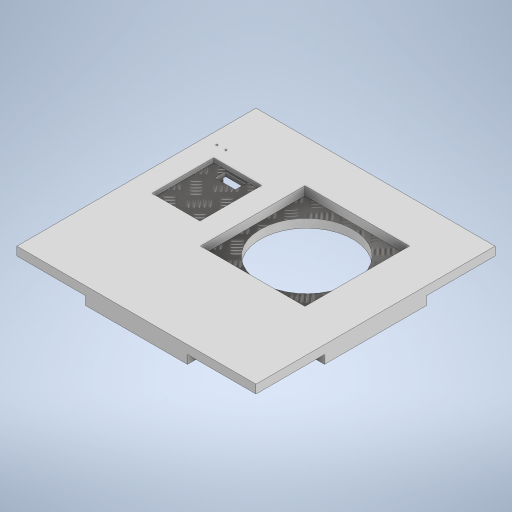
# Autodesk Inventor part: FinalBoxTop
Saved by Autodesk Inventor 2023 (Build 270158000, 158)
## iProperties
Created: 2023-09-21
Part Number: FinalBoxTop
Material: Generic
Document SubType Name: Modeling
Designer: Gage
Density: 1 g/cm^3
Appearance: Default
Author: Gage
## iProperties of the stored document FinalBoxTop_3DPrint.ipt
Created: 2023-09-28
Part Number: FinalBoxTop_3DPrint
Material: Generic
Document SubType Name: Modeling
Designer: Gage
Density: 1 g/cm^3
Appearance: Default
Author: Gage
Autodesk Inventor part; units mm, degrees
ref_plane "YZ Plane" through (0, 0, 0) normal (1, 0, 0) x (0, 1, 0)
ref_plane "XZ Plane" through (0, 0, 0) normal (0, 1, 0) x (-1, 0, 0)
ref_plane "XY Plane" through (0, 0, 0) normal (0, 0, 1) x (1, 0, 0)
sketch "Sketch1" plane through (0, 0, 0) normal (0, 1, 0) x (-1, 0, 0)
  line L0 (44.323, -44.323) -> (-44.323, -44.323)
  line L1 (-44.323, -44.323) -> (-44.323, 44.323)
  line L2 (-44.323, 44.323) -> (44.323, 44.323)
  line L3 (44.323, 44.323) -> (44.323, -44.323)
  point P0 (0, 0)
  point P1 (0, 44.323)
  point P2 (-44.323, 0)
  dimension "d0" = 88.646
  dimension "d1" = 88.646
  constraints: 8 end point, 2 midpoint, 2 parallel, 1 horizontal, 1 horizontal alignment, 1 perpendicular, 1 vertical alignment
  measures "d0" distance of L1.end L2.end
  measures "d1" distance of L0.end L1.end
extrude "Extrusion1" add sketch "Sketch1" along normal blind 6.35
sketch "Sketch2" plane through (0, 0, 0) normal (0, -1, 0) x (1, 0, 0)
  line L0 (-44.323, 44.323) -> (44.323, 44.323) projected
  line L1 (-44.323, 44.323) -> (-18.923, 44.323)
  line L2 (-18.923, 44.323) -> (-18.923, 18.923)
  line L3 (-18.923, 18.923) -> (-44.323, 18.923)
  line L4 (-44.323, 18.923) -> (-44.323, 44.323)
  line L5 (44.323, 44.323) -> (18.923, 44.323)
  line L6 (18.923, 44.323) -> (18.923, 18.923)
  line L7 (18.923, 18.923) -> (44.323, 18.923)
  line L8 (44.323, 18.923) -> (44.323, 44.323)
  line L9 (44.323, 44.323) -> (44.323, -44.323) projected
  line L10 (44.323, -44.323) -> (18.923, -44.323)
  line L11 (18.923, -44.323) -> (18.923, -18.923)
  line L12 (18.923, -18.923) -> (44.323, -18.923)
  line L13 (44.323, -18.923) -> (44.323, -44.323)
  line L14 (44.323, -44.323) -> (-44.323, -44.323) projected
  line L15 (-44.323, -44.323) -> (-18.923, -44.323)
  line L16 (-18.923, -44.323) -> (-18.923, -18.923)
  line L17 (-18.923, -18.923) -> (-44.323, -18.923)
  line L18 (-44.323, -18.923) -> (-44.323, -44.323)
  line L19 (44.323, -44.323) -> (28.448, -44.323)
  line L20 (28.448, -44.323) -> (28.448, -28.448)
  line L21 (28.448, -28.448) -> (44.323, -28.448)
  line L22 (44.323, -28.448) -> (44.323, -44.323)
  line L23 (28.448, -28.448) -> (28.448, -18.923)
  line L24 (28.448, -28.448) -> (18.923, -28.575)
  point P0 (0, 0)
  point P1 (44.323, -18.923)
  dimension "d4" = 25.4
  dimension "d5" = 25.4
  dimension "d6" = 25.4
  dimension "d7" = 25.4
  dimension "d8" = 25.4
  dimension "d9" = 25.4
  dimension "d10" = 25.4
  dimension "d11" = 25.4
  dimension "d147" = 15.875
  dimension "d148" = 15.875
  constraints: 44 end point, 10 parallel, 6 perpendicular, 5 horizontal, 2 point on line
  measures "d4" distance of L2.end L3.end
  measures "d5" distance of L1.end L2.end
  measures "d6" distance of L7.end L6.end
  measures "d7" distance of L6.end L5.end
  measures "d8" distance of L11.end L12.end
  measures "d9" distance of L10.end L11.end
  measures "d10" distance of L17.end L16.end
  measures "d11" distance of L16.end L15.end
  measures "d147" distance of L20.end L21.end
  measures "d148" distance of L19.end L20.end
extrude "Extrusion2" cut sketch "Sketch2" against normal blind 3.175 contours L0 L2 L3 L4 | L0 L8 L7 L6 | L9 L21 L23 L12 | L9 L10 L20 L21 | L20 L10 L11 L24 | L14 L18 L17 L16
sketch "Sketch3" plane through (0, 6.35, 0) normal (0, 1, 0) x (1, 0, 0)
  line L0 (-45.72, 45.72) -> (45.72, 45.72)
  line L1 (45.72, 45.72) -> (45.72, -45.72)
  line L2 (45.72, -45.72) -> (-45.72, -45.72)
  line L3 (-45.72, -45.72) -> (-45.72, 45.72)
  point P0 (0, 0)
  point P1 (45.72, 0)
  point P2 (0, 45.72)
  dimension "d14" = 91.44
  dimension "d15" = 91.44
  constraints: 8 end point, 2 midpoint, 2 parallel, 1 horizontal, 1 horizontal alignment, 1 perpendicular, 1 vertical alignment
  measures "d14" distance of L1.end L2.end
  measures "d15" distance of L0.end L1.end
extrude "Extrusion3" [suppressed]
sketch "Sketch4" plane through (0, 3.175, 0) normal (0, -1, 0) x (1, 0, 0)
  circle A0 centre (-38.1, 38.1) radius 3.175
  circle A1 centre (38.1, 38.1) radius 3.175
  circle A2 centre (38.1, -38.1) radius 3.175
  circle A3 centre (-38.1, -38.1) radius 3.175
  line L0 (44.323, 44.323) -> (44.323, 18.923) projected
  line L1 (18.923, 44.323) -> (44.323, 44.323) projected
  line L2 (-44.323, 44.323) -> (-18.923, 44.323) projected
  line L3 (-44.323, 18.923) -> (-44.323, 44.323) projected
  line L4 (-44.323, -44.323) -> (-44.323, -18.923) projected
  line L5 (-18.923, -44.323) -> (-44.323, -44.323) projected
  line L6 (44.323, -18.923) -> (44.323, -44.323) projected
  line L7 (44.323, -44.323) -> (18.923, -44.323) projected
  point P0 (0, 0)
  point P1 (44.323, 31.623)
  point P2 (-31.623, 44.323)
  point P3 (-44.323, -31.623)
  point P4 (44.323, -31.623)
  point P5 (31.623, -44.323)
  dimension "d19" = 6.35
  dimension "d20" = 6.35
  dimension "d21" = 6.35
  dimension "d22" = 6.35
  dimension "d23" = 6.223
  dimension "d24" = 6.223
  dimension "d25" = 6.223
  dimension "d26" = 6.223
  dimension "d27" = 6.223
  dimension "d28" = 6.223
  dimension "d29" = 6.223
  dimension "d30" = 6.223
  constraints: 5 midpoint, 4 centre point
  measures "d19" diameter of A0
  measures "d20" diameter of A1
  measures "d21" diameter of A2
  measures "d22" diameter of A3
  measures "d23" horizontal distance of point (44.323, 31.623) A1.centre
  measures "d24" distance from line of L1 A1.centre
  measures "d25" vertical distance of point (-31.623, 44.323) A0.centre
  measures "d26" distance from line of L3 A0.centre
  measures "d27" horizontal distance of point (-44.323, -31.623) A3.centre
  measures "d28" distance from line of L5 A3.centre
  measures "d29" horizontal distance of point (44.323, -31.623) A2.centre
  measures "d30" vertical distance of point (31.623, -44.323) A2.centre
extrude "Extrusion4" [suppressed]
sketch "Sketch5" plane through (0, 9.525, 0) normal (0, 1, 0) x (1, 0, 0)
  line L0 (44.323, 44.323) -> (-44.323, 44.323) projected
  line L1 (44.323, 44.323) -> (28.448, 44.323)
  line L2 (28.448, 44.323) -> (28.448, 28.448)
  line L3 (28.448, 28.448) -> (44.323, 28.448)
  line L4 (44.323, 28.448) -> (44.323, 44.323)
  line L5 (28.448, 28.448) -> (-10.287, 28.448)
  line L6 (-10.287, 28.448) -> (-10.287, -10.287)
  line L7 (-10.287, -10.287) -> (28.448, -10.287)
  line L8 (28.448, -10.287) -> (28.448, 28.448)
  line L9 (-10.287, 28.448) -> (-1.397, 28.448)
  line L10 (-1.397, 28.448) -> (-1.397, 22.6515)
  line L11 (-4.4905, 19.558) -> (-10.287, 19.558)
  line L12 (-10.287, 19.558) -> (-10.287, 28.448)
  line L13 (28.448, 28.448) -> (19.558, 28.448)
  line L14 (19.558, 28.448) -> (19.558, 22.6515)
  line L15 (22.6515, 19.558) -> (28.448, 19.558)
  line L16 (28.448, 19.558) -> (28.448, 28.448)
  line L17 (28.448, -10.287) -> (19.558, -10.287)
  line L18 (19.558, -10.287) -> (19.558, -4.4905)
  line L19 (22.6515, -1.397) -> (28.448, -1.397)
  line L20 (28.448, -1.397) -> (28.448, -10.287)
  line L21 (-10.287, -10.287) -> (-1.397, -10.287)
  line L22 (-1.397, -10.287) -> (-1.397, -4.4905)
  line L23 (-4.4905, -1.397) -> (-10.287, -1.397)
  line L24 (-10.287, -1.397) -> (-10.287, -10.287)
  circle A0 centre (9.0805, 9.0805) radius 17.145
  point P0 (0, 0)
  point P1 (19.558, -10.287)
  point P2 (28.448, -1.397)
  point P3 (-1.397, 28.448)
  point P4 (-10.287, 19.558)
  point P5 (-1.397, -4.4905)
  point P6 (19.558, -4.4905)
  point P7 (22.6515, -1.397)
  point P8 (-1.397, 22.6515)
  point P9 (-4.4905, 19.558)
  point P10 (-4.4905, -1.397)
  point P11 (28.448, 9.0805)
  point P12 (9.0805, 28.448)
  point P13 (-10.287, 24.003)
  point P14 (-5.842, -10.287)
  point P15 (-7.3888, -1.397)
  point P16 (28.448, 24.003)
  point P17 (19.558, 24.003)
  dimension "d125" = 34.29
  dimension "d33" = 15.875
  dimension "d34" = 15.875
  dimension "d35" = 38.735
  dimension "d36" = 38.735
  dimension "d126" = 8.89
  dimension "d127" = 8.89
  dimension "d128" = 8.89
  dimension "d129" = 8.89
  dimension "d130" = 8.89
  dimension "d131" = 8.89
  dimension "d132" = 8.89
  dimension "d133" = 8.89
  constraints: 48 end point, 12 parallel, 6 horizontal, 6 midpoint, 6 perpendicular, 1 horizontal alignment, 1 point on line, 1 vertical alignment, 10 other
  measures "d33" distance of L3.end L2.end
  measures "d34" distance of L2.end L1.end
  measures "d35" distance of L7.end L6.end
  measures "d36" distance of L6.end L5.end
  measures "d126" distance between parallel lines of L5 L11
  measures "d127" distance from line of L10 point (-10.287, 24.003)
  measures "d128" vertical distance of point (-5.842, -10.287) point (-7.389, -1.397)
  measures "d129" distance between parallel lines of L6 L22
  measures "d130" distance between parallel lines of L17 L19
  measures "d131" distance between parallel lines of L18 L8
  measures "d132" distance of point (28.448, 24.003) point (19.558, 24.003)
  measures "d133" distance between parallel lines of L5 L15
extrude "Extrusion5" [suppressed]
sketch "Sketch7" plane through (0, 9.525, 0) normal (0, 1, 0) x (1, 0, 0)
  line L0 (44.323, -44.323) -> (44.323, 44.323) projected
  line L1 (44.323, 44.323) -> (28.448, 44.323)
  line L2 (28.448, 44.323) -> (28.448, 28.448)
  line L3 (28.448, 28.448) -> (44.323, 28.448)
  line L4 (44.323, 28.448) -> (44.323, 44.323)
  line L5 (28.448, 28.448) -> (-10.287, 28.448)
  line L6 (-10.287, 28.448) -> (-10.287, -10.287)
  line L7 (-10.287, -10.287) -> (28.448, -10.287)
  line L8 (28.448, -10.287) -> (28.448, 28.448)
  line L9 (-10.287, 28.448) -> (-1.397, 28.448)
  line L10 (-10.287, 19.558) -> (-10.287, 28.448)
  line L11 (28.448, 28.448) -> (19.558, 28.448)
  line L12 (28.448, 19.558) -> (28.448, 28.448)
  line L13 (28.448, -10.287) -> (19.558, -10.287)
  line L14 (28.448, -1.397) -> (28.448, -10.287)
  line L15 (-10.287, -10.287) -> (-1.397, -10.287)
  line L16 (-10.287, -1.397) -> (-10.287, -10.287)
  point P0 (0, 0)
  point P1 (-1.397, 28.448)
  dimension "d62" = 15.875
  dimension "d63" = 15.875
  dimension "d64" = 38.735
  dimension "d65" = 38.735
  constraints: 32 end point, 6 horizontal, 4 parallel, 2 perpendicular
  measures "d62" distance of L3.end L2.end
  measures "d63" distance of L1.end L2.end
  measures "d64" distance of L7.end L6.end
  measures "d65" distance of L6.end L5.end
extrude "Extrusion7" [suppressed]
sketch "Sketch9" plane through (0, 9.525, 0) normal (0, 1, 0) x (1, 0, 0)
  point P0 (0, 0)
sketch "Sketch11" plane through (0, 9.525, 0) normal (0, 1, 0) x (1, 0, 0)
  point P0 (0, 0)
sketch "Sketch12" plane through (0, 0, 0) normal (0, -1, 0) x (1, 0, 0)
  line L0 (18.923, -44.323) -> (-31.75, -44.323)
  line L1 (-31.75, -44.323) -> (-31.75, -42.545)
  line L2 (18.923, -55.245) -> (18.923, -44.323)
  line L3 (-31.75, -42.545) -> (16263.8032, -42.545)
  line L4 (16263.8032, -42.545) -> (16263.8032, -31.623)
  line L5 (16263.8032, -31.623) -> (-31.75, -31.623)
  line L6 (-31.75, -31.623) -> (-31.75, -42.545)
  line L7 (-44.323, -18.923) -> (-44.323, 18.923) projected
  line L8 (16263.8032, -31.623) -> (-44.323, -31.623)
  line L9 (-44.323, -31.623) -> (-44.323, -30.0228)
  line L10 (-44.323, -30.0228) -> (16263.8032, -30.0228)
  line L11 (16263.8032, -30.0228) -> (16263.8032, -31.623)
  line L12 (-18.923, 18.923) -> (-44.323, 18.923) projected
  line L13 (-44.323, -30.0228) -> (-42.7228, -30.0228)
  line L14 (-42.7228, -30.0228) -> (-42.7228, 18.923)
  line L15 (-42.7228, 18.923) -> (-44.323, 18.923)
  line L16 (-44.323, 18.923) -> (-44.323, -30.0228)
  line L17 (-42.7228, 18.923) -> (-31.7277, 18.923)
  line L18 (-31.7277, 18.923) -> (-31.7277, 180.443)
  line L19 (-31.7277, 180.443) -> (-42.7228, 180.443)
  line L20 (-42.7228, 180.443) -> (-42.7228, 18.923)
  line L21 (-18.923, 44.323) -> (18.923, 44.323) projected
  line L22 (-31.7277, 180.443) -> (-30.1275, 180.443)
  line L23 (-30.1275, 180.443) -> (-30.1275, 44.323)
  line L24 (-30.1275, 44.323) -> (-31.7277, 44.323)
  line L25 (-31.7277, 44.323) -> (-31.7277, 180.443)
  line L26 (18.923, 18.923) -> (18.923, 44.323) projected
  line L27 (-30.1275, 44.323) -> (18.923, 44.323)
  line L28 (18.923, 44.323) -> (18.923, 42.7228)
  line L29 (18.923, 42.7228) -> (-30.1275, 42.7228)
  line L30 (-30.1275, 42.7228) -> (-30.1275, 44.323)
  line L31 (18.923, 42.7228) -> (17.3228, 42.7228)
  line L32 (17.3228, 42.7228) -> (17.3228, 18.923)
  line L33 (17.3228, 18.923) -> (18.923, 18.923)
  line L34 (18.923, 18.923) -> (18.923, 42.7228)
  line L35 (44.323, 44.323) -> (44.323, -44.323) projected
  line L36 (17.3228, 18.923) -> (44.323, 18.923)
  line L37 (44.323, 18.923) -> (44.323, 180.443)
  line L38 (44.323, 180.443) -> (17.3228, 180.443)
  line L39 (17.3228, 180.443) -> (17.3228, 18.923)
  line L40 (28.448, -18.923) -> (44.323, -18.923) projected
  line L41 (44.323, 180.443) -> (42.7228, 180.443)
  line L42 (42.7228, 180.443) -> (42.7228, -18.923)
  line L43 (42.7228, -18.923) -> (44.323, -18.923)
  line L44 (44.323, -18.923) -> (44.323, 180.443)
  line L45 (42.7228, -18.923) -> (18.923, -18.923)
  line L46 (18.923, -18.923) -> (18.923, -24.2084)
  line L47 (18.923, -24.2084) -> (42.7228, -24.2084)
  line L48 (42.7228, -24.2084) -> (42.7228, -18.923)
  line L49 (18.923, -24.2084) -> (17.3228, -24.2084)
  line L50 (17.3228, -24.2084) -> (17.3228, -42.545)
  line L51 (17.3228, -42.545) -> (18.923, -42.545)
  line L52 (18.923, -42.545) -> (18.923, -24.2084)
  line L53 (18.923, -44.323) -> (18.923, -28.575) projected
  line L54 (-18.923, -18.923) -> (-18.923, -44.323) projected
  line L55 (18.923, -44.323) -> (-18.923, -44.323)
  line L56 (-18.923, -44.323) -> (-18.923, -42.7228)
  line L57 (-18.923, -42.7228) -> (18.923, -42.7228)
  line L58 (18.923, -42.7228) -> (18.923, -44.323)
  line L59 (17.3228, -42.545) -> (18.923, -42.545)
  line L60 (18.923, -42.545) -> (18.923, -42.7228)
  line L61 (18.923, -42.7228) -> (17.3228, -42.7228)
  line L62 (17.3228, -42.7228) -> (17.3228, -42.545)
  line L63 (16263.8032, -42.545) -> (-18.923, -42.545)
  line L64 (-18.923, -42.545) -> (-18.923, -42.7228)
  line L65 (-18.923, -42.7228) -> (16263.8032, -42.7228)
  line L66 (16263.8032, -42.7228) -> (16263.8032, -42.545)
  line L67 (-10.287, -28.448) -> (28.448, -28.448) projected
  line L68 (-9.525, 9.525) -> (28.448, 9.525)
  line L69 (28.448, 9.525) -> (28.448, -28.448)
  line L70 (28.448, -28.448) -> (-9.525, -28.448)
  line L71 (-9.525, -28.448) -> (-9.525, 9.525)
  line L72 (17.3228, -24.2084) -> (-5.867, -24.2084)
  line L73 (-5.867, -24.2084) -> (-5.867, 154.3887)
  line L74 (-5.867, 154.3887) -> (17.3228, 154.3887)
  line L75 (17.3228, 154.3887) -> (17.3228, -24.2084)
  line L76 (17.3228, -24.2084) -> (-1.1916, -42.7228)
  line L77 (17.3228, -24.2084) -> (49.6283, -24.2084) construction
  line L78 (-1.1916, -42.7228) -> (-19.7059, -24.2084)
  line L79 (-1.1916, -42.7228) -> (35.5335, -42.7228) construction
  line L80 (-19.7059, -24.2084) -> (-32.8283, -42.7228)
  line L81 (-32.8283, -42.7228) -> (-42.7228, -35.7099)
  line L82 (-42.7228, -35.7099) -> (12.8674, 42.7228)
  line L83 (12.8674, 42.7228) -> (42.7228, 63.8728)
  line L84 (42.7228, 63.8728) -> (17.3228, 28.0357)
  line L85 (17.3228, 28.0357) -> (42.7228, 10.0331)
  line L86 (42.7228, 10.0331) -> (17.3228, -25.8039)
  line L87 (17.4453, -24.2084) -> (-2.7918, -42.7228)
  line L88 (-2.7918, -42.7228) -> (-19.7301, -24.2084)
  line L89 (-19.7301, -24.2084) -> (-39.9672, -42.7228)
  line L90 (-39.9672, -42.7228) -> (-42.7228, -39.7108)
  line L91 (-42.7228, -39.7108) -> (39.9672, 35.94)
  line L92 (39.9672, 35.94) -> (42.7228, 32.928)
  line L93 (42.7228, 32.928) -> (17.3228, 9.6902)
  line L94 (17.3228, 9.6902) -> (42.7228, -1.0828)
  line L95 (42.7228, -1.0828) -> (17.3228, -24.3205)
  line L96 (17.3228, -42.7228) -> (17.1896, -24.2084)
  line L97 (17.1896, -24.2084) -> (4.3578, -42.7228)
  line L98 (4.3578, -42.7228) -> (-22.3557, -24.2084)
  line L99 (-22.3557, -24.2084) -> (-35.0642, -42.545)
  line L100 (-42.545, -42.545) -> (42.545, -42.545) projected
  line L101 (-35.0642, -42.545) -> (16263.8032, -11338.832)
  line L102 (16263.8032, -11338.832) -> (-5.867, -34813.5541)
  line L103 (-5.867, -34813.5541) -> (-42.7228, -34788.0104)
  line L104 (-42.7228, -34788.0104) -> (24192.9295, 180.443)
  line L105 (42.7228, -24.2084) -> (17.3228, -17.3228)
  line L106 (17.3228, -17.3228) -> (42.7228, 76.3738)
  line L107 (42.7228, 76.3738) -> (17.3228, 83.2595)
  line L108 (17.3228, 83.2595) -> (42.7228, 176.9561)
  line L109 (42.7228, 176.9561) -> (29.8603, 180.443)
  line L110 (29.8603, 180.443) -> (22.7974, 154.3887)
  line L111 (42.7228, -22.6082) -> (17.3228, -15.7226)
  line L112 (17.3228, -15.7226) -> (42.7228, 77.974)
  line L113 (42.7228, 77.974) -> (17.3228, 84.8597)
  line L114 (17.3228, 84.8597) -> (42.7228, 22.3774)
  line L115 (42.7228, 22.3774) -> (431.5533, 180.443)
  line L116 (431.5533, 180.443) -> (442.1447, 154.3887)
  line L117 (15.7226, -42.7228) -> (15.5894, -24.2084)
  line L118 (15.5894, -24.2084) -> (-2558.3431, -42.7228)
  line L119 (-2558.3431, -42.7228) -> (-2558.4763, -24.2084)
  line L120 (-2558.4763, -24.2084) -> (-5132.4088, -42.7228)
  line L121 (-5132.4088, -42.7228) -> (-5095.6192, -5157.3332)
  line L122 (-5095.6192, -5157.3332) -> (-5.867, -5120.7225)
  line L123 (-5.867, -5120.7225) -> (-42.7228, 3.0988)
  line L124 (-42.7228, 3.0988) -> (5465.9431, 42.7228)
  line L125 (24192.9295, 180.443) -> (5046.5957, 42.7228)
  line L126 (5046.5957, 42.7228) -> (22.7974, 154.3887)
  line L127 (442.1447, 154.3887) -> (5465.9431, 42.7228)
  line L128 (-5.867, 154.3887) -> (-42.545, -32.2271)
  line L129 (-42.545, 42.545) -> (-42.545, -42.545) projected
  line L130 (-42.545, -32.2271) -> (-42.7228, -33.1317)
  line L131 (-42.7228, -33.1317) -> (-42.7228, -31.5315)
  line L132 (-42.7228, -31.5315) -> (6.1315, 42.7228)
  line L133 (-5.867, 154.3887) -> (-79.3356, 42.7228)
  line L134 (17.3228, -42.545) -> (16263.8032, -42.545)
  line L135 (-42.545, -30.0228) -> (-42.545, 180.443)
  point P0 (0, 0)
  point P1 (18.923, -18.923)
  point P2 (19.558, -28.448)
  point P3 (17.3228, -15.7226)
  point P4 (17.7269, -15.8321)
  point P5 (24.5726, -17.6879)
  point P6 (41.9227, -16.5227)
  point P7 (27.6372, 20.7253)
  point P8 (23.8906, 6.9046)
  point P9 (23.3165, -17.3474)
  point P10 (23.2233, -18.9223)
  point P11 (27.2733, 20.9832)
  point P12 (35.5727, 2.5273)
  point P13 (17.7269, 84.7501)
  point P14 (36.3728, 3.3274)
  point P15 (41.9227, 8.8773)
  point P16 (36.3728, 14.4272)
  point P17 (23.5015, 7.0696)
  point P18 (42.3187, 76.4834)
  point P19 (36.3728, 1.7272)
  point P20 (30.8229, -3.8227)
  point P21 (37.1729, 2.5273)
  point P22 (37.1729, 15.2273)
  point P23 (34.0995, 29.4005)
  point P24 (28.5496, 23.8506)
  point P25 (36.3728, 16.0274)
  point P26 (41.9227, 21.5773)
  point P27 (27.7495, 23.0505)
  point P28 (29.6259, 54.5948)
  point P29 (14.2544, 38.1458)
  point P30 (9.6774, 42.7228)
  point P31 (15.0545, 37.3457)
  point P32 (27.7495, 24.6507)
  point P33 (14.2544, 36.5456)
  point P34 (2.2571, 24.5482)
  point P35 (15.0079, 11.9091)
  point P36 (26.9494, 23.8506)
  point P37 (1.4535, 25.3448)
  point P38 (13.4543, 37.3457)
  point P39 (8.8773, 41.9227)
  point P40 (-3.1437, 29.9017)
  point P41 (-3.9474, 30.6982)
  point P42 (-42.545, 30.2006)
  point P43 (-42.545, 17.8544)
  point P44 (-4.7439, 29.9017)
  point P45 (-16.8706, 41.9221)
  point P46 (-41.7927, 16.7387)
  point P47 (-29.9115, 4.7341)
  point P48 (-24.5621, -0.6708)
  point P49 (0.6569, 24.5482)
  point P50 (-3.9403, 29.1051)
  point P51 (-29.1155, 3.9299)
  point P52 (-42.545, -21.6196)
  point P53 (-42.545, -35.4591)
  point P54 (-42.4465, -35.32)
  point P55 (1.4605, 23.7516)
  point P56 (-23.7661, -1.475)
  point P57 (-42.545, -31.2613)
  point P58 (-38.1458, -14.2544)
  point P59 (-42.545, -39.9051)
  point P60 (-37.3457, -13.4543)
  point P61 (-42.4764, -31.157)
  point P62 (-42.4169, -39.4309)
  point P63 (-40.2587, -37.4564)
  point P64 (-24.7626, -27.6376)
  point P65 (-37.3457, -15.0545)
  point P66 (-42.4714, -31.8526)
  point P67 (-36.5456, -14.2544)
  point P68 (-23.9584, -26.8416)
  point P69 (-11.7974, -14.8056)
  point P70 (17.1913, -24.4408)
  point P71 (30.0228, -30.0228)
  point P72 (18.4536, -24.2084)
  point P73 (17.3228, -25.8039)
  point P74 (22.3651, -18.6897)
  point P75 (17.3215, -42.545)
  point P76 (17.1906, -24.3406)
  point P77 (15.7213, -42.545)
  point P78 (15.6018, -25.9294)
  point P79 (-1.0138, -42.545)
  point P80 (15.6016, -25.8952)
  point P81 (15.6059, -26.4936)
  point P82 (10.8738, -36.2738)
  point P83 (-1.9561, -41.9583)
  point P84 (4.4811, -42.545)
  point P85 (-2.9544, -42.545)
  point P86 (10.0695, -37.0697)
  point P87 (-19.4539, -24.4605)
  point P88 (-20.8618, -25.2438)
  point P89 (-21.9659, -24.4786)
  point P90 (-19.4992, -24.4608)
  point P91 (-19.7165, -24.2233)
  point P92 (-20.5788, -25.4399)
  point P93 (2.8416, -42.545)
  point P94 (-2.5569, -37.2025)
  point P95 (-32.7022, -42.545)
  point P96 (-40.1298, -42.545)
  point P97 (-15.3311, -37.0691)
  point P98 (-22.5598, -42.545)
  point P99 (-30.2464, -34.9382)
  point P100 (-24.0131, -28.3871)
  point P101 (-29.4444, -33.8754)
  point P102 (-21.5341, -41.8678)
  point P103 (-16.0619, -36.3383)
  point P104 (-23.2172, -27.5828)
  point P105 (-15.266, -35.534)
  point P106 (-3.3612, -36.4066)
  point P107 (-9.0118, -30.8147)
  point P108 (-34.4103, -41.6015)
  point P109 (-36.8508, -39.8717)
  dimension "d94" = 1.6002
  dimension "d95" = 1.6002
  dimension "d96" = 1.6002
  dimension "d97" = 1.6002
  dimension "d98" = 1.6002
  dimension "d99" = 1.6002
  dimension "d100" = 1.6002
  dimension "d101" = 1.6002
  dimension "d102" = 135
  dimension "d103" = 135
  dimension "d104" = 1.6002
  dimension "d105" = 1.6002
  dimension "d106" = 1.6002
  dimension "d107" = 1.6002
  dimension "d108" = 1.6002
  dimension "d109" = 1.6002
  dimension "d110" = 1.6002
  constraints: 240 end point, 46 perpendicular, 42 point on line, 31 parallel, 22 horizontal, 3 vertical, 49 other
  measures "d94" distance of L8.end L9.end
  measures "d95" distance of L15.end L14.end
  measures "d96" distance of L24.end L23.end
  measures "d97" distance of L27.end L28.end
  measures "d98" distance of L33.end L32.end
  measures "d99" distance of L43.end L43.start
  measures "d100" distance of L51.end L50.end
  measures "d101" distance of L55.end L56.end
  measures "d102" angle of L76 L77
  measures "d103" angle of L79 L78
  measures "d104" distance of L87.start L86.end
  measures "d105" distance of L87.end L76.end
  measures "d106" distance of point (17.323, -15.723) L105.end
  measures "d107" distance of L111.start L47.end
  measures "d108" distance of L117.end L96.end
  measures "d109" distance of L117.start L61.end
  measures "d110" distance of L130.end L131.end
extrude "Extrusion10" [suppressed]
sketch "Sketch13" plane through (0, 9.525, 0) normal (0, 1, 0) x (1, 0, 0)
  circle A0 centre (-39.6875, -28.575) radius 0.3175
  circle A1 centre (-36.3855, -28.575) radius 0.3175
  line L0 (-45.72, 45.72) -> (-45.72, -45.72) projected
  line L1 (-45.72, -45.72) -> (45.72, -45.72) projected
  point P0 (0, 0)
  dimension "d113" = 0.635
  dimension "d114" = 0.635
  dimension "d115" = 3.302
  dimension "d149" = 6.0325
  dimension "d150" = 17.145
  constraints: 2 centre point
  measures "d113" diameter of A0
  measures "d114" diameter of A1
  measures "d115" distance of A1.centre A0.centre
  measures "d149" distance from line of L0 A0.centre
  measures "d150" distance from line of L1 A0.centre
extrude "Extrusion11" [suppressed]
sketch "Sketch14" plane through (0, 0, 0) normal (0, -1, 0) x (1, 0, 0)
  line L0 (-44.323, 44.323) -> (44.45, 44.323)
  line L1 (44.45, 44.323) -> (44.45, -44.45)
  line L2 (44.45, -44.45) -> (-44.323, -44.45)
  line L3 (-44.323, -44.45) -> (-44.323, 44.323)
  line L4 (14.2113, 11.1125) -> (-11.1786, 11.1125) projected
  line L5 (23.6397, -36.4059) -> (30.0228, -30.0228) projected
  line L6 (-11.1786, 11.1125) -> (30.0228, 11.1125)
  line L7 (30.0228, 11.1125) -> (30.0228, -30.0228)
  line L8 (30.0228, -30.0228) -> (-11.1786, -30.0228)
  line L9 (-11.1786, -30.0228) -> (-11.1786, 11.1125)
  point P0 (0, 0)
  constraints: 16 end point, 4 parallel, 2 horizontal, 2 perpendicular
extrude "Extrusion12" [suppressed]
fillet "Fillet3" [suppressed]
sketch "Sketch15" plane through (0, 6.35, 0) normal (0, 1, 0) x (1, 0, 0)
  line L0 (44.323, 44.323) -> (-44.323, 44.323) projected
  line L1 (44.323, 44.323) -> (28.448, 44.323)
  line L2 (28.448, 44.323) -> (28.448, 28.448)
  line L3 (28.448, 28.448) -> (44.323, 28.448)
  line L4 (44.323, 28.448) -> (44.323, 44.323)
  line L5 (28.448, 28.448) -> (-9.652, 28.448)
  line L6 (-9.652, 28.448) -> (-9.652, -9.652)
  line L7 (-9.652, -9.652) -> (28.448, -9.652)
  line L8 (28.448, -9.652) -> (28.448, 28.448)
  circle A0 centre (9.398, 9.398) radius 17.145
  point P0 (0, 0)
  point P1 (-9.652, 9.398)
  point P2 (9.398, 28.448)
  dimension "d134" = 15.875
  dimension "d135" = 15.875
  dimension "d136" = 38.1
  dimension "d137" = 38.1
  dimension "d138" = 34.29
  constraints: 16 end point, 4 parallel, 2 horizontal, 2 midpoint, 2 perpendicular, 1 centre point, 1 horizontal alignment, 1 vertical alignment
  measures "d134" distance of L3.end L2.end
  measures "d135" distance of L2.end L1.end
  measures "d136" distance of L7.end L6.end
  measures "d137" distance of L6.end L5.end
  measures "d138" diameter of A0
extrude "Extrusion13" cut sketch "Sketch15" against normal blind 6.35 contours A0
sketch "Sketch16" plane through (0, 6.35, 0) normal (0, 1, 0) x (1, 0, 0)
  line L0 (44.323, 44.323) -> (-44.323, 44.323) projected
  line L1 (44.323, 44.323) -> (28.448, 44.323)
  line L2 (28.448, 44.323) -> (28.448, 28.448)
  line L3 (28.448, 28.448) -> (44.323, 28.448)
  line L4 (44.323, 28.448) -> (44.323, 44.323)
  line L5 (28.448, 28.448) -> (-10.287, 28.448)
  line L6 (-10.287, 28.448) -> (-10.287, -10.287)
  line L7 (-10.287, -10.287) -> (28.448, -10.287)
  line L8 (28.448, -10.287) -> (28.448, 28.448)
  point P0 (0, 0)
  dimension "d141" = 15.875
  dimension "d142" = 15.875
  dimension "d143" = 38.735
  dimension "d144" = 38.735
  constraints: 16 end point, 4 parallel, 2 horizontal, 2 perpendicular
  measures "d141" distance of L3.end L2.end
  measures "d142" distance of L2.end L1.end
  measures "d143" distance of L7.end L6.end
  measures "d144" distance of L6.end L5.end
extrude "Extrusion14" cut sketch "Sketch16" against normal blind 3.175 contours L8 L7 L6 L5
sketch "Sketch17" plane through (0, 6.35, 0) normal (0, 1, 0) x (1, 0, 0)
  circle A0 centre (-39.751, 25.273) radius 0.3175
  circle A1 centre (-36.449, 25.273) radius 0.3175
  line L0 (-44.323, 44.323) -> (-44.323, -44.323) projected
  line L1 (-44.323, -44.323) -> (44.323, -44.323) projected
  line L2 (44.323, 44.323) -> (-44.323, 44.323) projected
  circle A2 centre (-38.1, 38.1) radius 3.175 projected
  line L3 (-39.751, 25.273) -> (-36.449, 25.273)
  point P0 (0, 0)
  point P1 (-45.72, -45.72)
  point P2 (-38.1, 25.273)
  dimension "d151" = 0.635
  dimension "d152" = 0.635
  dimension "d153" = 3.302
  dimension "d160" = 19.05
  dimension "d161" = 6.223
  dimension "d162" = 6.223
  constraints: 2 centre point, 2 end point, 1 horizontal, 1 midpoint
  measures "d151" diameter of A0
  measures "d152" diameter of A1
  measures "d153" distance of L3.end L3.start
  measures "d160" distance from line of L2 L3.start
  measures "d161" distance from line of L0 A2.centre
  measures "d162" distance from line of L0 point (-38.1, 25.273)
extrude "Extrusion15" cut sketch "Sketch17" against normal through all contours A0 | A1
sketch "Sketch18" plane through (0, 6.35, 0) normal (0, 1, 0) x (1, 0, 0)
  line L0 (-36.195, 20.5105) -> (-18.415, 20.5105)
  line L1 (-18.415, 20.5105) -> (-18.415, -2.3495)
  line L2 (-18.415, -2.3495) -> (-36.195, -2.3495)
  line L3 (-36.195, -2.3495) -> (-36.195, 20.5105)
  line L4 (-44.323, 44.323) -> (-44.323, -44.323) projected
  line L5 (-10.287, 28.448) -> (28.448, 28.448) projected
  point P0 (0, 0)
  point P1 (-27.305, 15.875)
  point P2 (-14.2875, 9.0805)
  point P3 (-27.305, 20.5105)
  point P4 (-18.415, 9.0805)
  dimension "d158" = 17.78
  dimension "d159" = 22.86
  dimension "d163" = 17.018
  dimension "d164" = 19.3675
  constraints: 8 end point, 2 midpoint, 2 parallel, 1 horizontal, 1 horizontal alignment, 1 perpendicular, 1 vertical alignment
  measures "d158" distance of L1.end L2.end
  measures "d159" distance of L0.end L1.end
  measures "d163" distance from line of L4 point (-27.305, 15.875)
  measures "d164" distance from line of L5 point (-14.287, 9.081)
extrude "Extrusion16" cut sketch "Sketch18" against normal blind 1.524
sketch "Sketch19" plane through (0, 4.826, 0) normal (0, 1, 0) x (1, 0, 0)
  line L0 (-31.115, 19.8755) -> (-23.495, 19.8755)
  line L1 (-23.495, 19.8755) -> (-23.495, 15.8115)
  line L2 (-23.495, 15.8115) -> (-31.115, 15.8115)
  line L3 (-31.115, 15.8115) -> (-31.115, 19.8755)
  line L4 (-36.195, 20.5105) -> (-18.415, 20.5105) projected
  line L5 (-18.415, 20.5105) -> (-18.415, -2.3495) projected
  point P0 (0, 0)
  point P1 (-27.305, 12.7)
  point P2 (-27.305, 15.8115)
  dimension "d167" = 7.62
  dimension "d168" = 4.064
  dimension "d169" = 0.635
  dimension "d170" = 8.89
  constraints: 8 end point, 2 parallel, 1 horizontal, 1 midpoint, 1 perpendicular, 1 vertical alignment
  measures "d167" distance of L1.end L2.end
  measures "d168" distance of L0.end L1.end
  measures "d169" distance between parallel lines of L4 L0
  measures "d170" distance from line of L5 point (-27.305, 12.7)
extrude "Extrusion17" cut sketch "Sketch19" against normal through all
shell "Shell1" thickness 2.54 removed faces 1 at (-6.3077, 0, 27.3897)
body "Solid1"
